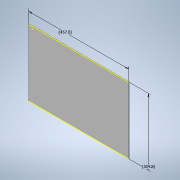
# Autodesk Inventor part: outerbox1plate
Saved by Autodesk Inventor 2021 (Build 250183000, 183)
## iProperties
Created: 2023-06-07
Part Number: outerbox1plate
Material: Generic
Document SubType Name: Modeling
Designer: badig
Density: 1 g/cm^3
Appearance: Default
Author: badig
Autodesk Inventor part; units mm, degrees
ref_plane "YZ Plane" through (0, 0, 0) normal (1, 0, 0) x (0, 1, 0)
ref_plane "XZ Plane" through (0, 0, 0) normal (0, 1, 0) x (-1, 0, 0)
ref_plane "XY Plane" through (0, 0, 0) normal (0, 0, 1) x (1, 0, 0)
sketch "Sketch1" plane through (0, 0, 0) normal (0, 0, 1) x (1, 0, 0)
  line L0 (-16.5031, 10.331) -> (441.2969, 10.331)
  line L1 (441.2969, 10.331) -> (441.2969, -294.469)
  line L2 (441.2969, -294.469) -> (-16.5031, -294.469)
  line L3 (-16.5031, -294.469) -> (-16.5031, 10.331)
  point P0 (0, 0)
  dimension "d0" = 457.8
  dimension "d1" = 304.8
  constraints: 8 end point, 2 parallel, 1 horizontal, 1 perpendicular
  measures "d0" distance of L1.end L2.end
  measures "d1" distance of L0.end L1.end
extrude "Extrusion1" add sketch "Sketch1" along normal blind 2
sketch "Sketch2" plane through (0, 0, 2) normal (0, 0, 1) x (1, 0, 0)
  line L0 (-16.5031, -294.469) -> (441.2969, -294.469) projected
  line L1 (441.2969, 10.331) -> (-16.5031, 10.331) projected
  point P0 (0, 0)
  dimension "d4" = 304.8
  dimension "d5" = 457.8
  measures "d4" distance between parallel lines of L0 L1
  measures "d5" distance of L1.start L1.end
body "Solid1"
